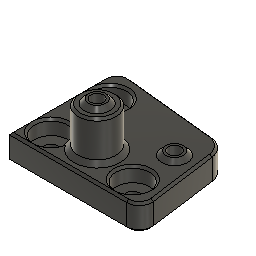
GT2_pulley_support_left_i2 v5 (Autodesk Fusion 360 design; units mm, degrees)
Autodesk Fusion 360 part; units mm, degrees
sketch "Sketch1" plane through (0, 0, 0) normal (0, 0, 1) x (1, 0, 0)
  circle A0 centre (-24.5, 5) radius 1.525
  circle A1 centre (-24.5, 5) radius 4
  circle A2 centre (-24.5, 15) radius 1.525
  line L0 (-31.5, 0) -> (-31.5, 26)
  line L1 (-31.5, 26) -> (0, 26)
  circle A3 centre (-14, 7) radius 1.525
  circle A4 centre (-5, 5) radius 1.525
  circle A5 centre (-5, 5) radius 4
  line L2 (-16.7, 5.4412) -> (-14, 3.8823)
  line L3 (-14, 3.8823) -> (-11.3, 5.4412)
  line L4 (-11.3, 5.4412) -> (-11.3, 8.5588)
  line L5 (-11.3, 8.5588) -> (-14, 10.1177)
  line L6 (-14, 10.1177) -> (-16.7, 8.5588)
  line L7 (-16.7, 8.5588) -> (-16.7, 5.4412)
  line L8 (-21.8, 16.5588) -> (-24.5, 18.1177)
  line L9 (-24.5, 18.1177) -> (-27.2, 16.5588)
  line L10 (-27.2, 16.5588) -> (-27.2, 13.4412)
  line L11 (-27.2, 13.4412) -> (-24.5, 11.8823)
  line L12 (-24.5, 11.8823) -> (-21.8, 13.4412)
  line L13 (-21.8, 13.4412) -> (-21.8, 16.5588)
  line L14 (-31.5, 0) -> (-28.886, 19.5909)
  line L15 (-31.5, 0) -> (-5.1135, 0) construction
  line L16 (0, 26) -> (-24.8803, 23.4728)
  line L17 (0, 26) -> (2, 26) construction
  arc A6 (-24.8803, 23.4728) -> (-28.886, 19.5909) centre (-24.4255, 18.9958) ccw
  circle A7 centre (-14, 7) radius 4.5
  line L18 (0, 0) -> (-31.5, 0)
  line L19 (-31.5, 0) -> (-31.5, 26)
  line L20 (-31.5, 26) -> (0, 26)
  line L21 (0, 26) -> (0, 0)
  circle A8 centre (-5, 19) radius 1.525
  circle A9 centre (-5, 19) radius 4
  line L22 (31.5, 0) -> (31.5, 26)
  arc A10 (28.886, 19.5909) -> (24.8803, 23.4728) centre (24.4255, 18.9958) ccw
  circle A11 centre (5, 19) radius 4
  circle A12 centre (5, 19) radius 1.525
  circle A13 centre (5, 5) radius 4
  circle A14 centre (5, 5) radius 1.525
  circle A15 centre (14, 7) radius 4.5
  circle A16 centre (14, 7) radius 1.525
  line L23 (16.7, 8.5588) -> (16.7, 5.4412)
  circle A17 centre (24.5, 5) radius 4
  circle A18 centre (24.5, 5) radius 1.525
  line L24 (27.2, 13.4412) -> (24.5, 11.8823)
  circle A19 centre (24.5, 15) radius 1.525
  line L25 (24.5, 11.8823) -> (21.8, 13.4412)
  line L26 (11.3, 8.5588) -> (14, 10.1177)
  line L27 (27.2, 16.5588) -> (27.2, 13.4412)
  line L28 (14, 10.1177) -> (16.7, 8.5588)
  line L29 (0, 26) -> (24.8803, 23.4728)
  line L30 (31.5, 0) -> (28.886, 19.5909)
  line L31 (0, 0) -> (31.5, 0)
  line L32 (16.7, 5.4412) -> (14, 3.8823)
  line L33 (14, 3.8823) -> (11.3, 5.4412)
  line L34 (11.3, 5.4412) -> (11.3, 8.5588)
  line L35 (21.8, 16.5588) -> (24.5, 18.1177)
  line L36 (24.5, 18.1177) -> (27.2, 16.5588)
  line L37 (21.8, 13.4412) -> (21.8, 16.5588)
  point P0 (-14, 7)
  point P1 (-24.5, 15)
  point P2 (14, 7)
  point P3 (24.5, 15)
  dimension "d5" = 3.05
  dimension "d6" = 8
  dimension "d7" = 3.05
  dimension "d11" = 3.05
  dimension "d12" = 3.05
  dimension "d13" = 8
  dimension "d24" = 2.7
  dimension "d25" = 2.7
  dimension "d28" = 82.4
  dimension "d29" = 174.2
  dimension "d31" = 4.5
  dimension "d51" = 9
  dimension "d52" = 31.5
  dimension "d53" = 26
  dimension "d54" = 5
  dimension "d55" = 14
  dimension "d56" = 24.5
  dimension "d57" = 24.5
  dimension "d58" = 5
  dimension "d59" = 5
  dimension "d60" = 7
  dimension "d61" = 15
  dimension "d62" = 3.05
  dimension "d63" = 19
  dimension "d64" = 5
  dimension "d65" = 8
  constraint concentric A0 A1
  constraint vertical L0
  constraint horizontal L1
  constraint concentric A4 A5
  constraint coincident P0 A3.centre
  constraint coincident P1 A2.centre
  constraint horizontal L15
  constraint horizontal L17
  constraint tangent L14 A6
  constraint tangent L16 A6
  constraint horizontal L18
  constraint vertical L19
  constraint horizontal L20
  constraint vertical L21
  constraint coincident L18.start L21.end
  constraint concentric A8 A9
  constraint symmetric A0 L21 A18
  constraint symmetric A1 L21 A17
  constraint symmetric A2 L21 A19
  constraint symmetric L0.start L21 L22.start
  constraint symmetric L1.end L21 L16.start
  constraint symmetric A3 L21 A16
  constraint symmetric A4 L21 A14
  constraint symmetric A5 L21 A13
  constraint symmetric L2.start L21 L23.end
  constraint symmetric L2.end L21 L32.end
  constraint symmetric L3.end L21 L33.end
  constraint symmetric L4.end L21 L26.start
  constraint symmetric L5.end L21 L26.end
  constraint symmetric L6.end L21 L23.start
  constraint symmetric P0 L21 P2
  constraint symmetric L8.start L21 L35.start
  constraint symmetric L8.end L21 L35.end
  constraint symmetric L9.end L21 L27.start
  constraint symmetric L10.end L21 L24.start
  constraint symmetric L11.end L21 L24.end
  constraint symmetric L12.end L21 L25.end
  constraint symmetric P1 L21 P3
  constraint symmetric L14.end L21 A10.start
  constraint symmetric L16.end L21 A10.end
  constraint symmetric A6 L21 A10
  constraint symmetric A7 L21 A15
  constraint symmetric L18.start L21 L31.start
  constraint symmetric L0.end L21 L22.end
  constraint symmetric L21 A8 A12
  constraint symmetric L21 A9 A11
  measures "d5" diameter of A0
  measures "d6" diameter of A1
  measures "d7" diameter of A2
  measures "d11" diameter of A3
  measures "d12" diameter of A4
  measures "d13" diameter of A5
  measures "d24" distance of P0 L7
  measures "d25" distance of P1 L13
  measures "d28" angle of L14 L15
  measures "d29" angle of L16 L17
  measures "d31" radius of A6
  measures "d51" diameter of A7
  measures "d52" distance of L18.start L0.start
  measures "d53" distance of L18.start L1.end
  measures "d54" horizontal distance of L18.start A4.centre
  measures "d55" horizontal distance of L18.start A3.centre
  measures "d56" horizontal distance of L18.start A0.centre
  measures "d57" horizontal distance of L18.start P1
  measures "d58" vertical distance of L18.start A0.centre
  measures "d59" vertical distance of L18.start A4.centre
  measures "d60" vertical distance of L18.start A3.centre
  measures "d61" vertical distance of L18.start P1
  measures "d62" diameter of A8
  measures "d63" vertical distance of L18.start A8.centre
  measures "d64" horizontal distance of L18.start A8.centre
  measures "d65" diameter of A9
extrude "Extrude7" add sketch "Sketch1" along normal blind 6 contours L21 A10 L29 L30 L31 | L24 L25 L27 L35 L36 L37
extrude "Extrude8" add sketch "Sketch1" along normal blind 15.5 contours A15 | L23 L26 L28 L32 L33 L34
extrude "Extrude9" add sketch "Sketch1" along normal blind 2.5 contours A11 | A13 | A17
extrude "Extrude10" cut sketch "Sketch1" along normal blind 2.5 contours L23 L26 L28 L32 L33 L34 | L24 L25 L27 L35 L36 L37
fillet "Fillet2" radius 3 2 edges at (0, 26, 3) (31.5, 0, 3)
sketch "Sketch4" plane through (0, 0, 15.5) normal (0, 0, 1) x (-1, 0, 0)
  circle A0 centre (-14, -7) radius 1.525
  circle A1 centre (-14, -7) radius 4.5
  circle A2 centre (-14, -7) radius 2.05
  dimension "d75" = 4.1
  constraint concentric A0 A2
  measures "d75" diameter of A2
extrude "Extrude11" add sketch "Sketch4" along normal blind 1 contours A2
chamfer "Chamfer5" distance 1 angle 45 1 edges at (15.9113, 6.2587, 15.5)
chamfer "Chamfer6" distance 1 angle 45 1 edges at (9.8045, 8.6273, 6)
sketch "Sketch5" plane through (0, 0, 6) normal (0, 0, 1) x (-1, 0, 0)
  arc A0 (-8.9908, -4.7289) -> (-8.5004, -6.9358) centre (-14, -7) ccw
  arc A1 (-8.5004, -6.9358) -> (-8.9908, -4.7289) centre (-5, -5) ccw
  circle A2 centre (-24.5, -5) radius 4
  circle A3 centre (-24.5, -15) radius 1.525
  circle A4 centre (-5, -19) radius 4
  arc A5 (-28.0731, 0) -> (-31.0468, -3.3968) centre (-28.0731, -3) ccw
  line L0 (-31.0468, -3.3968) -> (-28.886, -19.5909)
  arc A6 (-28.886, -19.5909) -> (-24.8803, -23.4728) centre (-24.4255, -18.9958) ccw
  line L1 (-24.8803, -23.4728) -> (-3.3032, -25.6645)
  arc A7 (-3.3032, -25.6645) -> (0, -22.6798) centre (-3, -22.6798) ccw
  line L2 (0, -22.6798) -> (0, 0)
  line L3 (0, 0) -> (-28.0731, 0)
  circle A8 centre (-24.5, -15) radius 2.05
  dimension "d80" = 4.1
  constraint concentric A3 A8
  measures "d80" diameter of A8
extrude "Extrude12" add sketch "Sketch5" along normal blind 1 contours A8
chamfer "Chamfer7" distance 1 angle 45 1 edges at (26.4113, 14.2587, 6)
chamfer "Chamfer8" distance 0.5 angle 45 18 edges at (1.2707, 20.4465, 6) (1.0953, 4.1323, 6) (9.8045, 5.3727, 15.5) (20.7707, 6.4465, 6) (14.0366, 0, 6) (30.3304, 1.0239, 6) (29.9664, 11.4939, 6) (27.5571, 22.2274, 6) (14.0917, 24.5686, 6) (0.9887, 24.9058, 6) (0, 11.3399, 6) (14.0366, 0, 0) (30.3304, 1.0239, 0) (29.9664, 11.4939, 0) (27.5571, 22.2274, 0) (14.0917, 24.5686, 0) (0.9887, 24.9058, 0) (0, 11.3399, 0)
equation "d24 = ( 5.4 / 2 ) * 1 mm"
equation "d25 = ( 5.4 / 2 ) * 1 mm"
